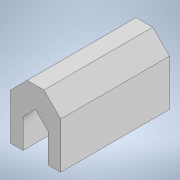
# Autodesk Inventor part: outside-join
Saved by Autodesk Inventor 2021 (Build 250183000, 183)
## iProperties
Created: 2020-12-08
Part Number: outside-join
Material: Generic
Document SubType Name: Modeling
Designer: Luke Kamols
Density: 1 g/cm^3
Appearance: Default
Author: Luke Kamols
Autodesk Inventor part; units mm, degrees
ref_plane "YZ Plane" through (0, 0, 0) normal (1, 0, 0) x (0, 1, 0)
ref_plane "XZ Plane" through (0, 0, 0) normal (0, 1, 0) x (-1, 0, 0)
ref_plane "XY Plane" through (0, 0, 0) normal (0, 0, 1) x (1, 0, 0)
sketch "Sketch1" plane through (0, 0, 0) normal (0, 0, 1) x (1, 0, 0)
  line L0 (3, 0) -> (6, 0)
  line L1 (6, 0) -> (6, 11)
  line L2 (0, 15) -> (2, 15)
  line L3 (2, 15) -> (6, 11)
  line L4 (0, 10) -> (3, 7)
  line L5 (3, 7) -> (3, 0)
  line L6 (-3, 0) -> (-6, 0)
  line L7 (-6, 0) -> (-6, 11)
  line L8 (0, 15) -> (-2, 15)
  line L9 (-2, 15) -> (-6, 11)
  line L10 (0, 10) -> (-3, 7)
  line L11 (-3, 7) -> (-3, 0)
  point P0 (0, 0)
  dimension "d1" = 3
  dimension "d2" = 11
  dimension "d4" = 2
  dimension "d5" = 10
  constraints: 24 end point, 1 perpendicular
  measures "d1" distance of L0.start L0.end
  measures "d2" distance of L0.end L1.end
  measures "d4" distance of L2.start L2.end
  measures "d5" distance of point (0, 0) L4.start
extrude "Extrusion1" add sketch "Sketch1" along normal blind 26
body "Solid1"
